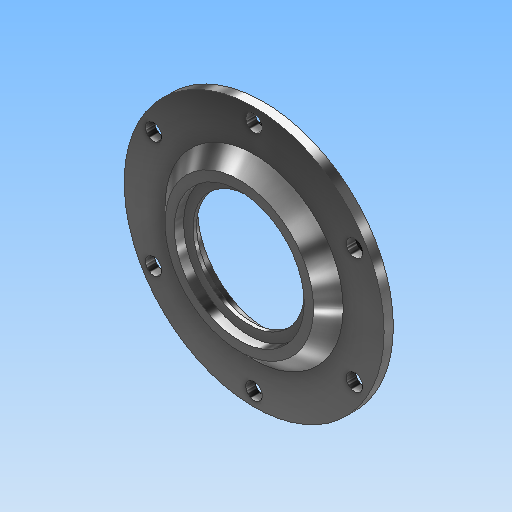
# Autodesk Inventor part: 7055-192 PART1
Saved by Autodesk Inventor 2020.1 (Build 241239000, 239)
## iProperties
Created: 2001-03-07
Part Number: 7055-192 PART1
Document SubType Name: Modeling
Designer: Joe M
Material: Steel, Mild
Engineer: Joe M
Density: 7.86 g/cm^3
Appearance: Chrome - Polished
Control State: 0
Master: False
Checked Out: False
Shininess: 20.0
Length Units: 11269
Angle Units: 11279
Time Units: 11290
Mass Units: 11283
Length Display Precision: 3
Angle Display Precision: 2
Compacted: True
Density: 0.0
Volumn: 0.0
Area: 0.0
PropertySet Name: Model Information
Author: Joe M
Autodesk Inventor part; units mm, degrees
ref_plane "YZ Plane" through (0, 0, 0) normal (1, 0, 0) x (0, 1, 0)
ref_plane "XZ Plane" through (0, 0, 0) normal (0, 1, 0) x (-1, 0, 0)
ref_plane "XY Plane" through (0, 0, 0) normal (0, 0, 1) x (1, 0, 0)
sketch "Sketch1" plane through (-195.9052, -159.4976, -9) normal (0, 0, 1) x (1, 0, 0)
  circle A0 centre (195.9052, 159.4976) radius 70
  dimension "d29" = 140
  constraints: 1 centre point, 1 other
  measures "d29" diameter of A0
extrude "ExtrusionBlind1" add sketch "Sketch1" along normal blind 18
sketch "Sketch2" plane through (-195.9052, -159.4976, -9) normal (0, 0, 1) x (1, 0, 0)
  circle A0 centre (195.9052, 159.4976) radius 55
  circle A1 centre (195.9052, 159.4976) radius 83.1126
  circle A2 centre (195.9052, 159.4976) radius 70 projected
  dimension "d30" = 166.2252
  dimension "d31" = 110
  constraints: 2 centre point, 1 coincident, 1 concentric
  measures "d30" diameter of A1
  measures "d31" diameter of A0
extrude "ExtrusionBlind2" cut sketch "Sketch2" along normal blind 5 contours A1 | A2
sketch "Sketch3" plane through (-195.9052, -159.4976, -9) normal (0, 0, 1) x (1, 0, 0)
  circle A0 centre (195.9052, 159.4976) radius 30
  circle A1 centre (195.9052, 159.4976) radius 55 projected
  dimension "d32" = 60
  constraints: 1 centre point, 1 concentric
  measures "d32" diameter of A0
extrude "ExtrusionThru1" cut sketch "Sketch3" along normal through all contours A0
sketch "Sketch4" plane through (-195.9052, -159.4976, -9) normal (0, 0, 1) x (1, 0, 0)
  circle A0 centre (195.9052, 159.4976) radius 37.5
  circle A1 centre (195.9052, 159.4976) radius 55 projected
  dimension "d33" = 75
  constraints: 1 centre point, 1 concentric
  measures "d33" diameter of A0
extrude "ExtrusionBlind3" cut sketch "Sketch4" along normal blind 11 contours A0
sketch "Sketch5" plane through (-195.9052, -159.4976, -9) normal (0, 0, 1) x (1, 0, 0)
  circle A0 centre (195.9052, 159.4976) radius 47.5
  circle A1 centre (195.9052, 159.4976) radius 55 projected
  dimension "d34" = 95
  constraints: 1 centre point, 1 concentric
  measures "d34" diameter of A0
extrude "ExtrusionBlind4" cut sketch "Sketch5" along normal blind 3 contours A0
sketch "Sketch6" plane through (0, 0, -4) normal (0, 0, -1) x (-1, 0, 0)
  point P0 (0, -62.5)
hole "Hole1" at (0, -62.5, -4) direction (0, 0, 1) diameter 9 end through all
pattern_circular "PolarArray1" count 6 over 360 about axis through (0, 0, -9) along (0, 0, -1) of "Hole1"
sketch "Sketch9" plane through (0, 0, 9) normal (0, 0, 1) x (1, 0, 0)
  circle A0 centre (0, 0) radius 35
  circle A1 centre (0, 0) radius 47.5 projected
  dimension "d35" = 70
  constraints: 3 other
  measures "d35" diameter of A0
extrude "ExtrusionBlind5" cut sketch "Sketch9" against normal blind 5 contours A0
sketch "Sketch10" plane through (0, 0, 9) normal (0, 0, 1) x (1, 0, 0)
  circle A0 centre (0, 0) radius 48
  circle A1 centre (0, 0) radius 87.5498
  circle A2 centre (0, 0) radius 55 projected
  dimension "d36" = 175.0996
  dimension "d37" = 96
  constraints: 5 other
  measures "d36" diameter of A1
  measures "d37" diameter of A0
extrude "ExtrusionBlind6" cut sketch "Sketch10" against normal blind 8 contours A1 | A2
chamfer "Chamfer1" distance 8 angle 45 1 edges at (-48, 0, 9)
body "Solid1"
